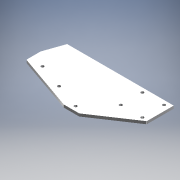
# Autodesk Inventor part: Sheet Metal Support Thing
Saved by Autodesk Inventor 2019.4 (Build 234330000, 330)
## iProperties
Created: 2020-01-11
Part Number: Sheet Metal Support Thing
Material: Aluminum 6061
Document SubType Name: Modeling
Designer: Mark
Mass: 226.139 g
Surface Area: 368.207 cm^2
Volume: 83.755 cm^3
Density: 2.7 g/cm^3
Appearance: Aluminum - Flat
Author: Mark
Autodesk Inventor part; units mm, degrees
ref_plane "YZ Plane" through (0, 0, 0) normal (1, 0, 0) x (0, 1, 0)
ref_plane "XZ Plane" through (0, 0, 0) normal (0, 1, 0) x (-1, 0, 0)
ref_plane "XY Plane" through (0, 0, 0) normal (0, 0, 1) x (1, 0, 0)
sketch "Sketch5" plane through (0, 0, 0) normal (0, 1, 0) x (-1, 0, 0)
  line L0 (0, 0) -> (150, 0)
  line L1 (150, 0) -> (150, -50)
  line L2 (150, -50) -> (0, -50)
  line L3 (0, -50) -> (0, 0)
  line L4 (30, -8.5) -> (124.4147, -41.4526) construction
  line L5 (30, -8.5) -> (130, -8.5) construction
  circle A0 centre (30, -8.5) radius 2.75
  circle A1 centre (124.4147, -41.4526) radius 2.75
  circle A2 centre (77.2073, -24.9763) radius 2.75
  line L6 (150, -37.1471) -> (43.627, 0)
  line L7 (150, -50) -> (-60, -50)
  line L8 (-60, -50) -> (-60, -100)
  line L9 (-60, -100) -> (150, -100)
  line L10 (150, -100) -> (150, -50)
  line L11 (-60, -50) -> (15, 0)
  line L12 (150, -50) -> (-60, -50)
  dimension "d22" = 150
  dimension "d23" = 50
  dimension "d26" = 100
  dimension "d27" = 19.24
  dimension "d28" = 5.5
  dimension "d29" = 5.5
  dimension "d30" = 5.5
  dimension "d31" = 8.5
  dimension "d32" = 30
  dimension "d33" = 19.25
  dimension "d34" = 12.5
  dimension "d35" = 210
  dimension "d36" = 50
  dimension "d37" = 15
  constraints: 26 end point, 4 horizontal, 4 parallel, 3 centre point, 3 point on line, 2 coincident, 2 perpendicular, 1 equal length, 1 midpoint
  measures "d22" distance of L1.end L2.end
  measures "d23" distance of L0.end L1.end
  measures "d26" distance of L4.start L4.end
  measures "d27" angle of L4 L5
  measures "d28" diameter of A0
  measures "d29" diameter of A1
  measures "d30" diameter of A2
  measures "d31" distance from line of L0 L4.start
  measures "d32" distance from line of L3 L4.start
  measures "d33" angle of L0 L6
  measures "d34" distance from line of L4.end L6
  measures "d35" distance of L9.end L8.end
  measures "d36" distance of L8.end L7.end
  measures "d37" distance of L0.start L11.end
extrude "Extrusion4" add sketch "Sketch5" along normal blind 5 contours L0 L11 L3 | L0 L6 L1 L2 L3 L11 | L3 L7 L11
sketch "Sketch6" plane through (0, 0, 0) normal (0, -1, 0) x (1, 0, 0)
  line L0 (60, -50) -> (-150, -50) projected
  line L1 (-150, -50) -> (60, -50)
  line L2 (60, -50) -> (60, -100)
  line L3 (60, -100) -> (-150, -100)
  line L4 (-150, -100) -> (-150, -50)
  point P0 (0, 0)
  dimension "d38" = 210
  dimension "d39" = 50
  constraints: 8 end point, 2 parallel, 1 horizontal, 1 perpendicular
  measures "d38" distance of L2.end L3.end
  measures "d39" distance of L1.end L2.end
extrude "Extrusion5" add sketch "Sketch6" against normal blind 5
sketch "Sketch7" plane through (0, 0, 0) normal (0, -1, 0) x (1, 0, 0)
  line L0 (0, -10) -> (60, -50) projected
  line L1 (0, -10) -> (-31.3138, 10.8759)
  line L2 (-43.627, 0) -> (0, 0) projected
  line L3 (-15, 0) -> (0, 0)
  line L4 (0, 0) -> (0, -10)
  constraints: 6 end point, 1 collinear, 1 horizontal, 1 perpendicular, 1 point on line
extrude "Extrusion6" cut sketch "Sketch7" against normal blind 5
fillet "Fillet1" radius 2 4 edges at (-150, 2.5, -37.1471) (-43.627, 2.5, 0) (-15, 2.5, 0) (60, 2.5, -50)
sketch "Sketch8" plane through (0, 0, 0) normal (0, -1, 0) x (1, 0, 0)
  line L0 (-150, -63.6277) -> (-0.7405, -11.5039)
  line L1 (-148.6594, -36.6789) -> (-43.9472, -0.1118) projected
  line L2 (-150, -63.6277) -> (-137.2982, -100)
  line L3 (60, -100) -> (-150, -100) projected
  line L4 (-137.2982, -100) -> (-150, -100)
  line L5 (-150, -100) -> (-150, -38.5671) projected
  line L6 (-150, -100) -> (-150, -63.6277)
  line L7 (50, -92) -> (10, -92) construction
  line L8 (10, -92) -> (10, -52) construction
  line L9 (10, -52) -> (50, -52) construction
  line L10 (50, -52) -> (50, -92) construction
  line L11 (50, -92) -> (10, -52) construction
  line L12 (10, -92) -> (50, -52) construction
  line L13 (60, -51.0704) -> (60, -100) projected
  circle A0 centre (10, -92) radius 2.75
  circle A1 centre (10, -52) radius 2.75
  circle A2 centre (50, -52) radius 2.75
  circle A3 centre (50, -92) radius 2.75
  point P0 (0, 0)
  point P1 (30, -72)
  dimension "d45" = 25
  dimension "d46" = 90
  dimension "d49" = 40
  dimension "d50" = 40
  dimension "d51" = 10
  dimension "d52" = 8
  dimension "d53" = 5.5
  dimension "d54" = 5.5
  dimension "d55" = 5.5
  dimension "d56" = 5.5
  constraints: 20 end point, 4 centre point, 4 coincident, 3 parallel, 2 horizontal, 2 midpoint, 2 point on line, 1 perpendicular, 1 vertical
  measures "d45" distance between parallel lines of L1 L0
  measures "d46" angle of L0 L2
  measures "d49" distance of L8.end L9.end
  measures "d50" distance of L7.end L8.end
  measures "d51" distance between parallel lines of L13 L10
  measures "d52" distance between parallel lines of L3 L7
  measures "d53" diameter of A0
  measures "d54" diameter of A1
  measures "d55" diameter of A2
  measures "d56" diameter of A3
extrude "Extrusion7" cut sketch "Sketch8" against normal blind 10
fillet "Fillet2" radius 2 2 edges at (-150, 2.5, -63.6277) (-137.2982, 2.5, -100)
body "Solid3"
